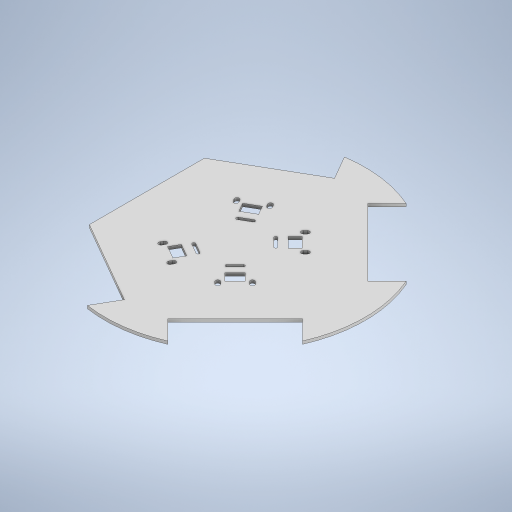
# Autodesk Inventor part: BaseV7
Saved by Autodesk Inventor 2024 (Build 280153000, 153)
## iProperties
Created: 2023-11-20
Part Number: BaseV7
Material: Generic
Document SubType Name: Modeling
Designer: felip
Density: 1 g/cm^3
Appearance: Default
Author: felip
Autodesk Inventor part; units mm, degrees
ref_plane "YZ Plane" through (0, 0, 0) normal (1, 0, 0) x (0, 1, 0)
ref_plane "XZ Plane" through (0, 0, 0) normal (0, 1, 0) x (-1, 0, 0)
ref_plane "XY Plane" through (0, 0, 0) normal (0, 0, 1) x (1, 0, 0)
sketch "Sketch1" plane through (0, 0, 0) normal (0, 1, 0) x (-1, 0, 0)
  line L0 (0, 0) -> (32.5, -56.2917)
  line L1 (0, 0) -> (90, 0) construction
  line L2 (0, 0) -> (35.5, 61.4878)
  line L3 (0, 0) -> (90, 0) construction
  line L4 (0, 0) -> (-50.2046, -50.2046)
  line L5 (0, 0) -> (90, 0) construction
  line L6 (0, 0) -> (-45.9619, 45.9619)
  line L7 (0, 0) -> (90, 0) construction
  line L8 (32.5, -56.2917) -> (13.95, -24.1621)
  line L9 (13.95, -24.1621) -> (16.45, -28.4922)
  line L10 (16.45, -28.4922) -> (20.7801, -25.9922)
  line L11 (16.45, -28.4922) -> (12.1199, -30.9922)
  line L12 (20.7801, -25.9922) -> (12.1199, -30.9922)
  line L13 (12.1199, -30.9922) -> (8.6199, -24.9301)
  line L14 (8.6199, -24.9301) -> (17.2801, -19.9301)
  line L15 (17.2801, -19.9301) -> (20.7801, -25.9922)
  line L16 (13.95, -24.1621) -> (17.7, -30.6573)
  line L17 (17.7, -30.6573) -> (10.3388, -34.9073)
  line L18 (17.7, -30.6573) -> (25.0612, -26.4073)
  line L19 (10.3388, -34.9073) -> (9.3388, -33.1752)
  line L20 (25.0612, -26.4073) -> (24.0612, -24.6752)
  circle A0 centre (25.0612, -26.4073) radius 1.5
  circle A1 centre (24.0612, -24.6752) radius 1.5
  circle A2 centre (10.3388, -34.9073) radius 1.5
  circle A3 centre (9.3388, -33.1752) radius 1.5
  line L21 (10.6378, -32.4252) -> (11.6378, -34.1573)
  line L22 (9.0397, -35.6573) -> (8.0397, -33.9252)
  line L23 (25.3603, -23.9252) -> (26.3603, -25.6573)
  line L24 (22.7622, -25.4252) -> (23.7622, -27.1573)
  line L25 (12.95, -22.4301) -> (9.95, -17.2339)
  line L26 (9.95, -17.2339) -> (14.2801, -14.7339)
  line L27 (9.95, -17.2339) -> (5.6199, -19.7339)
  line L28 (14.2801, -14.7339) -> (5.6199, -19.7339) construction
  line L29 (12.9141, -14.3679) -> (5.9859, -18.3679)
  line L30 (6.9859, -20.0999) -> (13.9141, -16.0999)
  arc A4 (13.9141, -16.0999) -> (12.9141, -14.3679) centre (13.4141, -15.2339) ccw
  arc A5 (5.9859, -18.3679) -> (6.9859, -20.0999) centre (6.4859, -19.2339) ccw
  line L31 (0, 0) -> (9.45, 16.3679)
  line L32 (16.45, 28.4922) -> (20.7801, 25.9922)
  line L33 (25.0612, 26.4073) -> (24.0612, 24.6752)
  line L34 (22.7622, 25.4252) -> (23.7622, 27.1573)
  line L35 (13.95, 24.1621) -> (17.7, 30.6573)
  line L36 (17.7, 30.6573) -> (25.0612, 26.4073)
  line L37 (20.7801, 25.9922) -> (17.2801, 19.9301)
  line L38 (16.45, 28.4922) -> (12.1199, 30.9922)
  line L39 (12.1199, 30.9922) -> (20.7801, 25.9922)
  circle A6 centre (24.0612, 24.6752) radius 1.5
  circle A7 centre (25.0612, 26.4073) radius 1.5
  line L40 (26.3603, 25.6573) -> (25.3603, 23.9252)
  line L41 (13.95, 24.1621) -> (16.45, 28.4922)
  line L42 (17.2801, 19.9301) -> (8.6199, 24.9301)
  line L43 (12.95, 22.4301) -> (9.95, 17.2339)
  arc A8 (12.9141, 14.3679) -> (13.9141, 16.0999) centre (13.4141, 15.2339) ccw
  line L44 (9.95, 17.2339) -> (14.2801, 14.7339)
  line L45 (13.9141, 16.0999) -> (6.9859, 20.0999)
  line L46 (9.95, 17.2339) -> (5.6199, 19.7339)
  arc A9 (6.9859, 20.0999) -> (5.9859, 18.3679) centre (6.4859, 19.2339) ccw
  line L47 (5.6199, 19.7339) -> (14.2801, 14.7339) construction
  line L48 (5.9859, 18.3679) -> (12.9141, 14.3679)
  line L49 (8.6199, 24.9301) -> (12.1199, 30.9922)
  line L50 (17.7, 30.6573) -> (10.3388, 34.9073)
  line L51 (10.3388, 34.9073) -> (9.3388, 33.1752)
  circle A10 centre (10.3388, 34.9073) radius 1.5
  circle A11 centre (9.3388, 33.1752) radius 1.5
  line L52 (10.6378, 32.4252) -> (11.6378, 34.1573)
  line L53 (8.0397, 33.9252) -> (9.0397, 35.6573)
  arc A12 (-10.5359, 16.1927) -> (-11.9501, 17.607) centre (-11.243, 16.8999) ccw
  line L54 (-14.0714, 14.0714) -> (-10.5359, 17.607)
  line L55 (-18.3141, 18.3141) -> (-14.0714, 14.0714)
  line L56 (-11.9501, 17.607) -> (-17.607, 11.9501)
  line L57 (-16.1927, 10.5359) -> (-10.5359, 16.1927)
  line L58 (-17.607, 10.5359) -> (-10.5359, 17.607) construction
  line L59 (-14.0714, 14.0714) -> (-17.607, 10.5359)
  arc A13 (-17.607, 11.9501) -> (-16.1927, 10.5359) centre (-16.8999, 11.243) ccw
  line L60 (-23.2638, 23.2638) -> (-19.7283, 26.7993)
  line L61 (-19.7283, 19.7283) -> (-25.0316, 25.0316)
  line L62 (-19.7283, 26.7993) -> (-14.7785, 21.8496)
  line L63 (-26.7993, 19.7283) -> (-19.7283, 26.7993)
  line L64 (-19.7283, 19.7283) -> (-23.2638, 23.2638)
  line L65 (-23.2638, 23.2638) -> (-26.7993, 19.7283)
  line L66 (-28.5671, 18.6676) -> (-29.9813, 20.0818)
  line L67 (-25.0316, 25.0316) -> (-31.042, 19.0212)
  line L68 (-31.042, 19.0212) -> (-29.6278, 17.607)
  circle A14 centre (-31.042, 19.0212) radius 1.5
  line L69 (-30.6884, 16.5463) -> (-32.1026, 17.9605)
  circle A15 centre (-29.6278, 17.607) radius 1.5
  line L70 (-21.8496, 14.7785) -> (-26.7993, 19.7283)
  line L71 (-14.7785, 21.8496) -> (-21.8496, 14.7785)
  line L72 (-19.0212, 31.042) -> (-17.607, 29.6278)
  line L73 (-18.6676, 28.5671) -> (-20.0818, 29.9813)
  circle A16 centre (-17.607, 29.6278) radius 1.5
  line L74 (-17.9605, 32.1026) -> (-16.5463, 30.6884)
  circle A17 centre (-19.0212, 31.042) radius 1.5
  line L75 (-25.0316, 25.0316) -> (-19.0212, 31.042)
  line L76 (-32.1026, -17.9605) -> (-30.6884, -16.5463)
  line L77 (-31.042, -19.0212) -> (-29.6278, -17.607)
  circle A18 centre (-29.6278, -17.607) radius 1.5
  line L78 (-28.5671, -18.6676) -> (-29.9813, -20.0818)
  circle A19 centre (-31.042, -19.0212) radius 1.5
  line L79 (-25.0316, -25.0316) -> (-31.042, -19.0212)
  line L80 (-19.7283, -19.7283) -> (-25.0316, -25.0316)
  line L81 (-19.7283, -26.7993) -> (-26.7993, -19.7283)
  line L82 (-14.7785, -21.8496) -> (-19.7283, -26.7993)
  line L83 (-23.2638, -23.2638) -> (-19.7283, -26.7993)
  line L84 (-25.0316, -25.0316) -> (-19.0212, -31.042)
  line L85 (-18.6676, -28.5671) -> (-20.0818, -29.9813)
  line L86 (-19.0212, -31.042) -> (-17.607, -29.6278)
  circle A20 centre (-17.607, -29.6278) radius 1.5
  circle A21 centre (-19.0212, -31.042) radius 1.5
  line L87 (-16.5463, -30.6884) -> (-17.9605, -32.1026)
  arc A22 (-16.1927, -10.5359) -> (-17.607, -11.9501) centre (-16.8999, -11.243) ccw
  line L88 (-14.0714, -14.0714) -> (-17.607, -10.5359)
  line L89 (-18.3141, -18.3141) -> (-14.0714, -14.0714)
  line L90 (-17.607, -11.9501) -> (-11.9501, -17.607)
  line L91 (-10.5359, -16.1927) -> (-16.1927, -10.5359)
  line L92 (-19.7283, -19.7283) -> (-23.2638, -23.2638)
  arc A23 (-11.9501, -17.607) -> (-10.5359, -16.1927) centre (-11.243, -16.8999) ccw
  line L93 (-21.8496, -14.7785) -> (-14.7785, -21.8496)
  line L94 (-14.0714, -14.0714) -> (-10.5359, -17.607)
  line L95 (-10.5359, -17.607) -> (-17.607, -10.5359) construction
  line L96 (-23.2638, -23.2638) -> (-26.7993, -19.7283)
  line L97 (-26.7993, -19.7283) -> (-21.8496, -14.7785)
  line L98 (35.5, -61.4878) -> (64.0788, -44.9878)
  line L99 (35.5, -61.4878) -> (6.9212, -77.9878)
  line L100 (64.0788, -44.9878) -> (70.4447, -56.0138)
  line L101 (6.9212, -77.9878) -> (13.287, -89.0138)
  line L102 (-50.2046, -50.2046) -> (-26.8701, -73.5391)
  line L103 (-50.2046, -50.2046) -> (-73.5391, -26.8701)
  line L104 (-73.5391, -26.8701) -> (-82.5418, -35.8727)
  line L105 (-26.8701, -73.5391) -> (-35.8727, -82.5418)
  line L106 (6.9212, 77.9878) -> (13.287, 89.0138)
  line L107 (35.5, 61.4878) -> (6.9212, 77.9878)
  line L108 (35.5, 61.4878) -> (64.0788, 44.9878)
  line L109 (64.0788, 44.9878) -> (70.4447, 56.0138)
  line L110 (-50.2046, 50.2046) -> (-73.5391, 26.8701)
  line L111 (-73.5391, 26.8701) -> (-82.5418, 35.8727)
  line L112 (-50.2046, 50.2046) -> (-26.8701, 73.5391)
  line L113 (-26.8701, 73.5391) -> (-35.8727, 82.5418)
  line L114 (64.0788, 44.9878) -> (64.0788, -44.9878)
  arc A24 (-35.8727, -82.5418) -> (13.287, -89.0138) centre (0, 0) ccw
  arc A25 (13.287, 89.0138) -> (-35.8727, 82.5418) centre (0, 0) ccw
  arc A26 (-82.5418, 35.8727) -> (-82.5418, -35.8727) centre (0, 0) ccw
  line L115 (35.5, 61.4878) -> (32.5, 56.2917)
  line L116 (64.0788, 44.9878) -> (61.0788, 39.7917)
  line L117 (6.9212, 77.9878) -> (3.9212, 72.7917)
  line L118 (3.9212, 72.7917) -> (32.5, 56.2917)
  line L119 (61.0788, 39.7917) -> (32.5, 56.2917)
  line L120 (64.0788, -44.9878) -> (61.0788, -39.7917)
  line L121 (61.0788, -39.7917) -> (3.9212, -72.7917)
  line L122 (3.9212, -72.7917) -> (6.9212, -77.9878)
  line L123 (-26.8701, -73.5391) -> (-22.6274, -69.2965)
  line L124 (-22.6274, -69.2965) -> (-69.2965, -22.6274)
  line L125 (-69.2965, -22.6274) -> (-73.5391, -26.8701)
  line L126 (-73.5391, 26.8701) -> (-69.2965, 22.6274)
  line L127 (-69.2965, 22.6274) -> (-22.6274, 69.2965)
  line L128 (-22.6274, 69.2965) -> (-26.8701, 73.5391)
  point P0 (9.95, -17.2339)
  point P1 (9.95, 17.2339)
  point P2 (-14.0714, 14.0714)
  point P3 (-13.3643, 13.3643)
  point P4 (-14.0714, -14.0714)
  point P5 (-13.3643, -13.3643)
  dimension "d43" = 43.1
  dimension "d44" = 5
  dimension "d45" = 5
  dimension "d46" = 5
  dimension "d47" = 7
  dimension "d48" = 7.5
  dimension "d49" = 8.5
  dimension "d50" = 8.5
  dimension "d51" = 2
  dimension "d52" = 2
  dimension "d53" = 3
  dimension "d54" = 3
  dimension "d55" = 3
  dimension "d56" = 3
  dimension "d57" = 6
  dimension "d58" = 5
  dimension "d59" = 2
  dimension "d76" = 18.9
  dimension "d79" = 120
  dimension "d83" = 75
  dimension "d87" = 90
  dimension "d89" = 33
  dimension "d90" = 33
  dimension "d92" = 33
  dimension "d96" = 120
  dimension "d100" = 90
  dimension "d104" = 6
  dimension "d105" = 6
  dimension "d106" = 6
  dimension "d107" = 6
  constraints: 266 end point, 62 point on circle, 27 centre point, 26 point on line, 16 coincident, 12 perpendicular, 6 tangent, 4 horizontal, 4 midpoint, 4 parallel, 2 collinear, 1 vertical, 211 other
  measures "d43" distance of L98.start L8.end
  measures "d44" distance of L8.end L9.end
  measures "d45" distance of L9.end L10.end
  measures "d46" distance of L9.end L11.end
  measures "d47" distance of L11.end L13.end
  measures "d48" distance of L8.end L16.end
  measures "d49" distance of L16.end L17.end
  measures "d50" distance of L16.end L18.end
  measures "d51" distance of L17.end L19.end
  measures "d52" distance of L18.end L20.end
  measures "d53" diameter of A0
  measures "d54" diameter of A1
  measures "d55" diameter of A2
  measures "d56" diameter of A3
  measures "d57" distance of L25.start L25.end
  measures "d58" distance of L25.end L27.end
  measures "d59" diameter of A5
  measures "d76" distance of L0.start L31.end
  measures "d89" distance of L98.start L98.end
  measures "d90" distance of L98.start L99.end
  measures "d92" distance of L4.end L102.end
  measures "d104" distance of L2.end L115.end
  measures "d105" distance of L108.end L116.end
  measures "d106" distance of L106.start L117.end
  measures "d107" distance of L102.end L123.end
extrude "Extrusion1" add sketch "Sketch1" along normal blind 2 contours L14 L13 L11 L0 L121 L122 L101 A24 L105 L123 L124 L4 L81 L82 L93 L90 A23 L91 L29 A5 L30 | L0 L30 A4 L29 L2 L48 A8 L45 L42 L37 L32 L119 L116 L114 L120 L121 L10 L15 L14 | L121 L120 L98 L99 L122 | L6 L57 A12 L56 L71 L62 L60 L127 L128 L113 A25 L106 L117 L118 L2 L38 L49 L42 L45 A9 L48 | L4 L91 A22 L90 L93 L97 L81 L124 L125 L104 A26 L111 L126 L127 L6 L63 L70 L71 L56 A13 L57 | L116 L119 L2 L108 | L2 L118 L117 L107 | L102 L4 L124 L123 | L103 L125 L124 L4 | L128 L127 L126 L110 L112
sketch "Sketch2" plane through (0, 2, 0) normal (0, 1, 0) x (1, 0, 0)
  line L0 (-6.9212, -77.9878) -> (-13.287, -89.0138) projected
  line L1 (-13.287, -89.0138) -> (-6.9212, -77.9878)
  line L2 (-6.9212, -77.9878) -> (-3.9212, -72.7917)
  line L3 (-3.9212, -72.7917) -> (-61.0788, -39.7917)
  line L4 (-61.0788, -39.7917) -> (-64.0788, -44.9878)
  line L5 (-6.9212, 77.9878) -> (-64.0788, 44.9878) projected
  line L6 (-13.1717, 88.814) -> (-6.9212, 77.9878)
  line L7 (-6.9212, 77.9878) -> (-3.9212, 72.7917)
  line L8 (-3.9212, 72.7917) -> (-61.0788, 39.7917)
  line L9 (-61.0788, 39.7917) -> (-64.0788, 44.9878)
  line L10 (26.8701, 73.5391) -> (35.8727, 82.5418) projected
  line L11 (26.8701, 73.5391) -> (22.6274, 69.2965)
  line L12 (22.6274, 69.2965) -> (69.2965, 22.6274)
  line L13 (69.2965, 22.6274) -> (73.5391, 26.8701)
  line L14 (73.5391, -26.8701) -> (69.2965, -22.6274)
  line L15 (69.2965, -22.6274) -> (22.6274, -69.2965)
  line L16 (22.6274, -69.2965) -> (26.8701, -73.5391)
  line L17 (35.8727, -82.5418) -> (26.8701, -73.5391) projected
  line L18 (26.8701, -73.5391) -> (73.5391, -26.8701)
  line L19 (73.5391, 26.8701) -> (26.8701, 73.5391)
  line L20 (-6.9212, 77.9878) -> (-64.0788, 44.9878)
  line L21 (-64.0788, -44.9878) -> (-6.9212, -77.9878)
  line L22 (-61.0788, -39.7917) -> (-61.0788, 39.7917)
  line L23 (-64.0788, 44.9878) -> (-64.0788, -44.9878)
  point P0 (0, 0)
  dimension "d108" = 6
  dimension "d109" = 66
  dimension "d110" = 6
  dimension "d111" = 66
  dimension "d112" = 6
  constraints: 40 end point, 11 perpendicular, 3 collinear, 2 point on line, 1 parallel, 1 vertical
  measures "d108" distance of L0.start L2.end
  measures "d109" distance of L2.end L3.end
  measures "d110" distance of L10.start L11.end
  measures "d111" distance of L11.end L12.end
  measures "d112" distance of L14.start L14.end
extrude "Extrusion2" cut sketch "Sketch2" against normal blind 2
body "Solid1"
